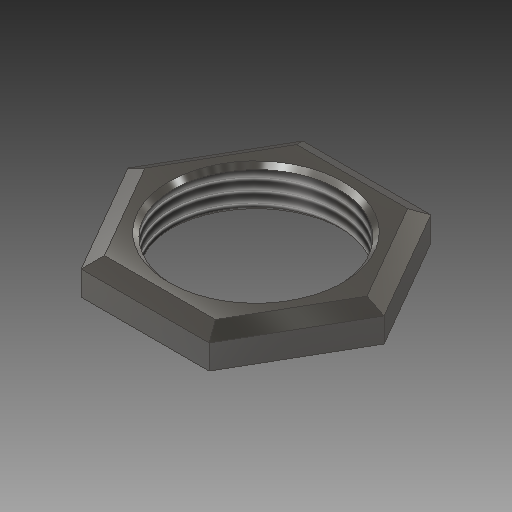
# Autodesk Inventor part: гайка
Saved by Autodesk Inventor 2019 (Build 230136000, 136)
## iProperties
Created: 2019-07-16
Part Number: гайка
Material: Сталь, нержавеющая, полированная
Document SubType Name: Modeling
Designer: Boss
Mass: 1.90279 g
Surface Area: 3.79556 cm^2
Volume: 0.237849 cm^3
Density: 8 g/cm^3
Appearance: Нержавеющая — полированная
Author: Boss
Autodesk Inventor part; units mm, degrees
ref_plane "YZ Plane" through (0, 0, 0) normal (1, 0, 0) x (0, 1, 0)
ref_plane "XZ Plane" through (0, 0, 0) normal (0, 1, 0) x (-1, 0, 0)
ref_plane "XY Plane" through (0, 0, 0) normal (0, 0, 1) x (1, 0, 0)
sketch "Эскиз1" plane through (0, 0, 0) normal (0, 1, 0) x (-1, 0, 0)
  line L0 (-4.3301, -7.5) -> (-8.6603, 0)
  line L1 (-8.6603, 0) -> (-4.3301, 7.5)
  line L2 (-4.3301, 7.5) -> (4.3301, 7.5)
  line L3 (4.3301, 7.5) -> (8.6603, 0)
  line L4 (8.6603, 0) -> (4.3301, -7.5)
  line L5 (4.3301, -7.5) -> (-4.3301, -7.5)
  circle A0 centre (0, 0) radius 5.6
  dimension "d0" = 15
  dimension "d1" = 11.2
  constraints: 12 end point, 2 coincident, 1 centre point, 1 horizontal, 13 other
  measures "d0" distance between parallel lines of L2 L5
  measures "d1" diameter of A0
extrude "Выдавливание1" add sketch "Эскиз1" along normal blind 2.8
chamfer "Фаска1" distance 1 angle 30 6 edges at (0, 2.8, 7.5) (6.4952, 2.8, 3.75) (6.4952, 2.8, -3.75) (0, 2.8, -7.5) (-6.4952, 2.8, -3.75) (-6.4952, 2.8, 3.75) measured on face at (0.225, 2.8, 6.8531)
chamfer "Фаска2" distance 1 angle 30 6 edges at (-6.4952, 0, 3.75) (0, 0, 7.5) (6.4952, 0, 3.75) (6.4952, 0, -3.75) (0, 0, -7.5) (-6.4952, 0, -3.75) measured on face at (0.225, 0, 6.8531)
thread "Резьба1" size "M12x0.75" class "6H" standard "ANSI Metric M Profile" full length
chamfer "Фаска3" distance 0.3 angle 45 2 edges at (5.6, 2.8, 0) (5.6, 0, 0)
